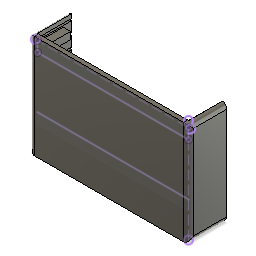
NixieGehaeuseObenUnten (Autodesk Fusion 360 design; units mm, degrees)
Autodesk Fusion 360 part; units mm, degrees
sketch "Skizze1" plane through (0, 0, 0) normal (0, 1, 0) x (1, 0, 0)
  line L0 (75, 35) -> (75, -35) construction
  line L1 (75, -35) -> (-75, -35) construction
  line L2 (-75, -35) -> (-75, 35) construction
  line L3 (-75, 35) -> (75, -35) construction
  line L4 (75, 35) -> (-75, -35) construction
  line L5 (73, 33) -> (73, -33) construction
  line L6 (73, -33) -> (-73, -33) construction
  line L7 (-73, -33) -> (-73, 33) construction
  line L8 (-73, 33) -> (73, -33) construction
  line L9 (73, 33) -> (-73, -33) construction
  line L10 (77, 37) -> (77, -37) construction
  line L11 (77, -37) -> (-77, -37) construction
  line L12 (-77, -37) -> (-77, 37) construction
  line L13 (-77, 37) -> (77, -37) construction
  line L14 (77, 37) -> (-77, -37) construction
  line L15 (-77, 0) -> (-77, -37)
  line L16 (-77, -37) -> (77, -37)
  line L17 (77, -37) -> (77, 0)
  line L18 (77, 0) -> (73, 0)
  line L19 (73, -33) -> (-73, -33)
  line L20 (-73, 0) -> (-73, -33)
  line L21 (-73, 0) -> (-77, 0)
  line L22 (73, 0) -> (73, -33)
  dimension "d1" = 150
  dimension "d2" = 70
  dimension "d3" = 146
  dimension "d4" = 66
  dimension "d5" = 154
  dimension "d6" = 74
  constraint parallel L0 L2
  constraint coincident L3 origin
  constraint coincident L4 origin
  constraint parallel L5 L7
  constraint coincident L8 origin
  constraint coincident L9 origin
  constraint parallel L10 L12
  constraint coincident L13 origin
  constraint coincident L14 origin
  constraint midpoint L12 L15.start
  constraint midpoint L10 L17.end
  constraint midpoint L5 L18.end
  constraint perpendicular L7 L19
  constraint midpoint L7 L20.start
  constraint perpendicular L19 L20
  measures "d1" distance of L0.end L1.end
  measures "d2" distance of L0.start L0.end
  measures "d3" distance of L5.end L6.end
  measures "d4" distance of L5.start L5.end
  measures "d5" distance of L10.end L11.end
  measures "d6" distance of L10.start L10.end
extrude "Extrusion1" add sketch "Skizze1" along normal blind 100 makes body 1
sketch "Skizze2" plane through (0, 0, 0) normal (0, 0, -1) x (-1, 0, 0)
  line L0 (-77, 0) -> (-73, 0)
  line L1 (-73, 0) -> (-73, 100)
  line L2 (-73, 100) -> (-77, 100)
  line L3 (-77, 100) -> (-77, 0)
  line L4 (-75, 12) -> (75, 12)
  line L5 (75, 12) -> (75, 10)
  line L6 (75, 10) -> (-75, 10)
  line L7 (-75, 10) -> (-75, 12)
  line L8 (-75, 24) -> (75.0643, 24)
  line L9 (75.0643, 24) -> (75.0643, 22)
  line L10 (75.0643, 22) -> (-75, 22)
  line L11 (-75, 22) -> (-75, 24)
  line L12 (-73, 0) -> (73, 0)
  line L13 (-75, 96) -> (75, 96)
  line L14 (75, 96) -> (75, 94)
  line L15 (75, 94) -> (-75, 94)
  line L16 (-75, 94) -> (-75, 96)
  line L17 (-73, 100) -> (73, 100)
  line L18 (75, 34) -> (-75, 34)
  line L19 (-75, 34) -> (-75, 36)
  line L20 (-75, 36) -> (75, 36)
  line L21 (75, 36) -> (75, 34)
  line L22 (75, 46) -> (-75, 46)
  line L23 (-75, 46) -> (-75, 48)
  line L24 (-75, 48) -> (75, 48)
  line L25 (75, 48) -> (75, 46)
  line L26 (75, 58) -> (-75, 58)
  line L27 (-75, 58) -> (-75, 60)
  line L28 (-75, 60) -> (75, 60)
  line L29 (75, 60) -> (75, 58)
  line L30 (75, 70) -> (-75, 70)
  line L31 (-75, 70) -> (-75, 72)
  line L32 (-75, 72) -> (75, 72)
  line L33 (75, 72) -> (75, 70)
  line L34 (75, 82) -> (-75, 82)
  line L35 (-75, 82) -> (-75, 84)
  line L36 (-75, 84) -> (75, 84)
  line L37 (75, 84) -> (75, 82)
  dimension "d11" = 10
  dimension "d12" = 2
  dimension "d14" = 2
  dimension "d45" = 2
  dimension "d46" = 2
  dimension "d47" = 2
  dimension "d48" = 2
  dimension "d49" = 2
  dimension "d50" = 10
  dimension "d51" = 10
  dimension "d52" = 10
  dimension "d53" = 10
  dimension "d54" = 10
  dimension "d55" = 2
  dimension "d57" = 10
  dimension "d59" = 4
  constraint horizontal L4
  constraint vertical L5
  constraint horizontal L6
  constraint vertical L7
  constraint horizontal L8
  constraint vertical L9
  constraint horizontal L10
  constraint vertical L11
  constraint horizontal L13
  constraint vertical L14
  constraint horizontal L15
  constraint vertical L16
  constraint horizontal L18
  constraint vertical L19
  constraint horizontal L20
  constraint vertical L21
  constraint horizontal L22
  constraint vertical L23
  constraint horizontal L24
  constraint vertical L25
  constraint horizontal L26
  constraint vertical L27
  constraint horizontal L28
  constraint vertical L29
  constraint horizontal L30
  constraint vertical L31
  constraint horizontal L32
  constraint vertical L33
  constraint horizontal L34
  constraint vertical L35
  constraint horizontal L36
  constraint vertical L37
  measures "d11" distance of L0 L6.end
  measures "d12" distance of L8 L10
  measures "d14" distance of L13 L15
  measures "d45" distance of L4 L6
  measures "d46" distance of L18.end L19.end
  measures "d47" distance of L22.end L23.end
  measures "d48" distance of L26.end L27.end
  measures "d49" distance of L30.end L31.end
  measures "d50" distance of L4 L10
  measures "d51" distance of L8 L18
  measures "d52" distance of L20 L22
  measures "d53" distance of L24 L26
  measures "d54" distance of L28 L30
  measures "d55" distance of L34.end L35.end
  measures "d57" distance of L32 L34
  measures "d59" distance of L13 L17
extrude "Extrusion4" cut sketch "Skizze2" against normal blind 35 contours L1 L4 L6 L7 | L1 L4 L5 L6 | L1 L13 L14 L15 | L1 L13 L15 L16 | L1 L8 L10 L11 | L1 L8 L9 L10 | L1 L34 L36 L37 | L1 L34 L35 L36 | L1 L18 L19 L20 | L1 L18 L20 L21 | L1 L30 L32 L33 | L1 L30 L31 L32 | L1 L22 L23 L24 | L1 L22 L24 L25 | L1 L26 L28 L29 | L1 L26 L27 L28 bodies 1
sketch "Skizze3" plane through (0, 0, 33) normal (0, 0, -1) x (-1, 0, 0)
  line L0 (-73, 24) -> (73, 24)
  line L1 (73, 24) -> (73, 34)
  line L2 (73, 94) -> (-73, 94)
  line L3 (-73, 34) -> (-73, 24)
  line L4 (-73, 0) -> (-73, 100) construction
  line L5 (75, 94) -> (-75, 94) construction
  line L6 (73, 34) -> (-73, 34)
  line L7 (-73, 84) -> (73, 84)
  line L8 (73, 84) -> (73, 94)
  line L9 (-73, 94) -> (-73, 84)
sketch "Skizze4" plane through (0, 0, 33) normal (0, 0, -1) x (-1, 0, 0)
  line L0 (-73, 93) -> (-66, 93)
  line L1 (-66, 93) -> (-66, 86)
  line L2 (-66, 86) -> (-73, 86)
  line L3 (-73, 86) -> (-73, 93)
  line L4 (-73, 13.9107) -> (-66, 13.9107)
  line L5 (-66, 13.9107) -> (-66, 20.9107)
  line L6 (-66, 20.9107) -> (-73, 20.9107)
  line L7 (-73, 20.9107) -> (-73, 13.9107)
  line L8 (73, 13.7285) -> (66, 13.7285)
  line L9 (66, 13.7285) -> (66, 20.7285)
  line L10 (66, 20.7285) -> (73, 20.7285)
  line L11 (73, 20.7285) -> (73, 13.7285)
  line L12 (72.9869, 92.6346) -> (65.9869, 92.6346)
  line L13 (65.9869, 92.6346) -> (65.9869, 85.6346)
  line L14 (65.9869, 85.6346) -> (72.9869, 85.6346)
  line L15 (72.9869, 85.6346) -> (72.9869, 92.6346)
  dimension "d29" = 7
  dimension "d30" = 7
  dimension "d33" = 7
  dimension "d34" = 7
  dimension "d35" = 7
  dimension "d36" = 7
  constraint horizontal L0
  constraint vertical L1
  constraint horizontal L2
  constraint vertical L3
  constraint horizontal L4
  constraint vertical L5
  constraint horizontal L6
  constraint vertical L7
  constraint horizontal L8
  constraint vertical L9
  constraint horizontal L10
  constraint vertical L11
  constraint horizontal L12
  constraint vertical L13
  constraint horizontal L14
  constraint vertical L15
  measures "d29" distance of L4.start L4.end
  measures "d30" distance of L4.start L6.end
  measures "d33" distance of L8.start L8.end
  measures "d34" distance of L8.start L10.end
  measures "d35" distance of L12.start L12.end
  measures "d36" distance of L12.start L14.end
extrude "Extrusion5" add sketch "Skizze4" along normal blind 25 separate body makes body 2 at (73, 18.5774, 24.6667) makes body 3 at (-68.3203, 85.6346, 24.6667) makes body 4 at (70.6667, 93, 24.6667) makes body 5 at (-66, 16.0618, 24.6667)
sketch "Skizze5" plane through (0, 0, 8) normal (0, 0, -1) x (-1, 0, 0)
  line L0 (-73, 86) -> (-66, 86)
  line L1 (-66, 86) -> (-66, 93)
  line L2 (-66, 93) -> (-73, 93)
  line L3 (-73, 93) -> (-73, 86)
  circle A0 centre (-69.5, 89.5) radius 2
  dimension "d39" = 4
  measures "d39" diameter of A0
sketch "Skizze6" plane through (0, 0, 8) normal (0, 0, -1) x (-1, 0, 0)
  line L0 (-73, 20.9107) -> (-73, 13.9107)
  line L1 (-73, 13.9107) -> (-66, 13.9107)
  line L2 (-66, 13.9107) -> (-66, 20.9107)
  line L3 (-66, 20.9107) -> (-73, 20.9107)
  circle A0 centre (-69.5, 17.4107) radius 2
  dimension "d40" = 4
  dimension "d61" = 3.5
  measures "d40" diameter of A0
  measures "d61" distance of L1 A0.centre
sketch "Skizze7" plane through (0, 0, 8) normal (0, 0, -1) x (-1, 0, 0)
  line L0 (73, 20.7285) -> (66, 20.7285)
  line L1 (66, 20.7285) -> (66, 13.7285)
  line L2 (66, 13.7285) -> (73, 13.7285)
  line L3 (73, 13.7285) -> (73, 20.7285)
  circle A0 centre (69.5, 17.2285) radius 2
  dimension "d60" = 3.5
  dimension "d64" = 4
  measures "d60" distance of L2 A0.centre
  measures "d64" diameter of A0
sketch "Skizze8" plane through (0, 0, 8) normal (0, 0, -1) x (-1, 0, 0)
  line L0 (72.9869, 85.6346) -> (72.9869, 92.6346)
  line L1 (72.9869, 92.6346) -> (65.9869, 92.6346)
  line L2 (65.9869, 92.6346) -> (65.9869, 85.6346)
  line L3 (65.9869, 85.6346) -> (72.9869, 85.6346)
  circle A0 centre (69.4869, 89.1346) radius 2
  dimension "d41" = 4
  measures "d41" diameter of A0
extrude "Extrusion6" cut sketch "Skizze8" sketch "Skizze7" sketch "Skizze6" sketch "Skizze5" against normal blind 25 contours A0 of sketch 2 contours A0 of sketch 3 contours A0 of sketch 4 contours A0 bodies 2 3 4 5
fillet "Abrundung1" radius 5 6 edges at (77, 50, 37) (-77, 50, 37) (-77, 0, 18.5) (77, 0, 18.5) (77, 100, 18.5) (-77, 100, 18.5) on bodies 1
